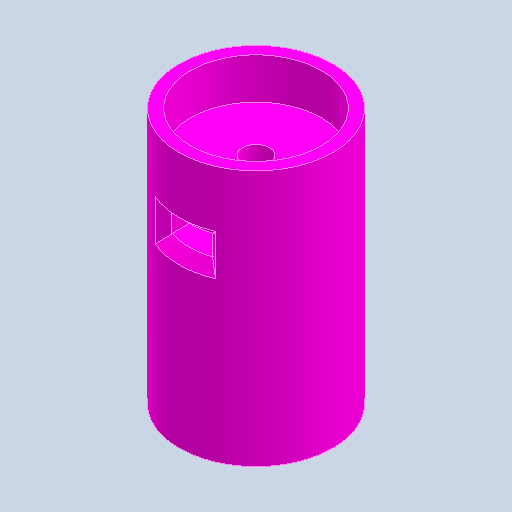
# Autodesk Inventor part: магнит_стойка
Saved by Autodesk Inventor 2023.1 (Build 271208000, 208)
## iProperties
Created: 2025-02-04
Part Number: магнит_стойка
Material: Типовые
Document SubType Name: Modeling
Designer: baranovaem
Density: 1 g/cm^3
Appearance: Пурпурный
Author: baranovaem
Autodesk Inventor part; units mm, degrees
ref_plane "YZ Plane" through (0, 0, 0) normal (1, 0, 0) x (0, 1, 0)
ref_plane "XZ Plane" through (0, 0, 0) normal (0, 1, 0) x (-1, 0, 0)
ref_plane "XY Plane" through (0, 0, 0) normal (0, 0, 1) x (1, 0, 0)
sketch "Эскиз1" plane through (0, 0, 0) normal (0, 1, 0) x (-1, 0, 0)
  circle A0 centre (0, 0) radius 15
  circle A1 centre (0, 0) radius 12.75
  dimension "d0" = 30
  dimension "d1" = 25.5
  constraints: 2 centre point, 2 coincident
  measures "d0" diameter of A0
  measures "d1" diameter of A1
extrude "Выдавливание1" add sketch "Эскиз1" along normal blind 50
sketch "Эскиз2" plane through (0, 0, 0) normal (0, -1, 0) x (1, 0, 0)
  circle A0 centre (0, 0) radius 15 projected
extrude "Выдавливание2" add sketch "Эскиз2" against normal blind 42
sketch "Эскиз3" plane through (0, 0, 0) normal (0, -1, 0) x (1, 0, 0)
  circle A0 centre (-5.5, -5) radius 1.25
  circle A1 centre (5.5, -5) radius 1.25
  circle A2 centre (-5.5, 5) radius 1.25
  circle A3 centre (5.5, 5) radius 1.25
  line L0 (5.5, 5) -> (-5.5, 5)
  line L1 (-5.5, 5) -> (-5.5, -5)
  line L2 (-5.5, -5) -> (5.5, -5)
  line L3 (5.5, -5) -> (5.5, 5)
  line L4 (5.5, -5) -> (-5.5, 5) construction
  point P0 (0, 0)
  point P1 (0, 0)
  dimension "d6" = 2.5
  dimension "d7" = 2.5
  dimension "d8" = 2.5
  dimension "d9" = 2.5
  constraints: 10 end point, 4 centre point, 3 coincident, 2 parallel, 1 horizontal, 1 midpoint, 1 perpendicular
  measures "d6" diameter of A0
  measures "d7" diameter of A1
  measures "d8" diameter of A2
  measures "d9" diameter of A3
extrude "Выдавливание3" cut sketch "Эскиз3" against normal blind 15 contours L2 L1 A0 | A0 L1 L2 | L2 L3 A1 | A1 L3 L2 | L1 L0 A2 | A2 L0 L1 | L3 L0 A3 | A3 L0 L3
sketch "Эскиз4" plane through (0, 42, 0) normal (0, 1, 0) x (1, 0, 0)
  circle A0 centre (0, 0) radius 2.65
  dimension "d12" = 5.3
  constraints: 1 centre point, 1 coincident
  measures "d12" diameter of A0
extrude "Выдавливание4" cut sketch "Эскиз4" against normal through all
sketch "Эскиз5" plane through (0, 0, 0) normal (0, 0, 1) x (1, 0, 0)
  line L0 (-4, 37) -> (4, 37)
  line L1 (4, 37) -> (4, 33)
  line L2 (4, 33) -> (-4, 33)
  line L3 (-4, 33) -> (-4, 37)
  line L4 (-4, 37) -> (4, 33) construction
  line L5 (4, 37) -> (-4, 33) construction
  point P0 (0, 0)
  point P1 (0, 35)
  dimension "d15" = 4
  dimension "d16" = 8
  constraints: 12 end point, 2 midpoint, 2 parallel, 1 horizontal, 1 perpendicular
  measures "d15" distance between parallel lines of L2 L0
  measures "d16" distance of L0.start L0.end
extrude "Выдавливание5" cut sketch "Эскиз5" along normal through all both and the other way through all
chamfer "Фаска1" distance 2 angle 45 8 edges at (0, 33, 15) (0, 33, -15) (-4, 35, 14.4568) (-4, 35, -14.4568) (0, 37, 15) (0, 37, -15) (4, 35, 14.4568) (4, 35, -14.4568)
